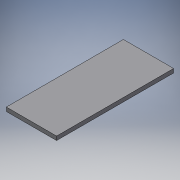
# Autodesk Inventor part: GearCoverTop
Saved by Autodesk Inventor 2019 (Build 230136000, 136)
## iProperties
Created: 2019-08-08
Part Number: GearCoverTop
Material: Generic
Document SubType Name: Modeling
Designer: aorfi
Density: 1 g/cm^3
Appearance: Default
Author: aorfi
Autodesk Inventor part; units mm, degrees
ref_plane "YZ Plane" through (0, 0, 0) normal (1, 0, 0) x (0, 1, 0)
ref_plane "XZ Plane" through (0, 0, 0) normal (0, 1, 0) x (-1, 0, 0)
ref_plane "XY Plane" through (0, 0, 0) normal (0, 0, 1) x (1, 0, 0)
sketch "Sketch1" plane through (0, 0, 0) normal (0, 1, 0) x (-1, 0, 0)
  line L0 (-13.8735, 30) -> (13.8735, 30)
  line L1 (13.8735, 30) -> (13.8735, -30)
  line L2 (13.8735, -30) -> (-13.8735, -30)
  line L3 (-13.8735, -30) -> (-13.8735, 30)
  line L4 (-13.8735, 30) -> (13.8735, -30) construction
  line L5 (13.8735, 30) -> (-13.8735, -30) construction
  point P0 (0, 0)
  dimension "d2" = 60
  dimension "d3" = 27.747
  constraints: 12 end point, 2 midpoint, 2 parallel, 1 horizontal, 1 perpendicular
  measures "d2" distance of L0.end L1.end
  measures "d3" distance of L1.end L2.end
extrude "Extrusion1" add sketch "Sketch1" along normal mid plane 2
sketch "Sketch2" plane through (0, 1, 0) normal (0, 1, 0) x (1, 0, 0)
  circle A0 centre (0, 0) radius 5
  dimension "d4" = 10
  constraints: 1 centre point, 1 coincident
  measures "d4" diameter of A0
extrude "Extrusion2" cut sketch "Sketch2" against normal through all
sketch "Sketch3" plane through (0, 1, 0) normal (0, 1, 0) x (1, 0, 0)
  line L0 (0, 0) -> (0, 30) construction
  line L1 (-13.8735, 30) -> (13.8735, 30) construction
  line L2 (0, 0) -> (0, -30) construction
  line L3 (13.8735, -30) -> (-13.8735, -30) construction
  point P0 (0, -15)
  point P1 (0, 15)
  constraints: 4 end point, 4 midpoint
hole "Hole1" at (0, 1, 15) at (0, 1, -15) direction (0, -1, 0) diameter 4.305 end through all clearance for "Flat Head Machine Screw (82)" size "#6" standard "Ansi Unified Screw Threads"
sketch "Sketch4" plane through (0, -1, 0) normal (0, -1, 0) x (1, 0, 0)
  circle A0 centre (-11.8735, 28) radius 0.965
  circle A1 centre (-11.8735, -28) radius 0.965
  circle A2 centre (11.8735, -28) radius 0.965
  circle A3 centre (11.8735, 28) radius 0.965
  line L0 (-13.8735, 30) -> (-13.8735, -30) projected
  line L1 (13.8735, 30) -> (-13.8735, 30) projected
  line L2 (13.8735, -30) -> (13.8735, 30) projected
  line L3 (-13.8735, -30) -> (13.8735, -30) projected
  point P0 (0, 0)
  dimension "d14" = 1.93
  dimension "d15" = 2
  dimension "d16" = 2
  dimension "d17" = 2
  dimension "d18" = 2
  constraints: 4 centre point, 3 equal radius, 2 horizontal alignment, 2 vertical alignment
  measures "d14" diameter of A0
  measures "d15" distance from line of L0 A0.centre
  measures "d16" distance from line of L1 A0.centre
  measures "d17" distance from line of L2 A3.centre
  measures "d18" distance from line of L3 A1.centre
extrude "Extrusion3" add sketch "Sketch4" along normal blind 2 contours A0 | A1 | A2 | A3
fillet "Fillet1" radius 2 4 edges at (13.8735, 0, 30) (-13.8735, 0, 30) (-13.8735, 0, -30) (13.8735, 0, -30)
equation "\"d16\" = d15"
equation "\"d17\" = d15"
equation "\"d18\" = d15"
body "Solid1"
